Autodesk Inventor part; units mm, degrees
(part 7 of 16)
  spline S39 degree 3 poles (-0.3054, 38.2473) (-0.3514, 38.3741) (-0.3956, 38.5015) (-0.4377, 38.6297) (-0.4605, 38.6989) (-0.4826, 38.7684) (-0.5042, 38.838) (-0.5246, 38.904) (-0.5444, 38.9701) (-0.5636, 39.0364) (-0.5817, 39.099) (-0.5993, 39.1617) (-0.6163, 39.2246) (-0.6323, 39.2837) (-0.6478, 39.3429) (-0.6627, 39.4023) (-0.6767, 39.458) (-0.6902, 39.5137) (-0.7032, 39.5696) (-0.7154, 39.6217) (-0.727, 39.6739) (-0.7382, 39.7262) (-0.7486, 39.7747) (-0.7586, 39.8232) (-0.7681, 39.8719) (-0.7769, 39.9168) (-0.7853, 39.9617) (-0.7932, 40.0067) (-0.8005, 40.0479) (-0.8075, 40.0891) (-0.814, 40.1304) (-0.82, 40.1679) (-0.8256, 40.2054) (-0.8309, 40.243) (-0.8357, 40.2767) (-0.8402, 40.3104) (-0.8443, 40.3442) (-0.8497, 40.3889) (-0.8545, 40.4336) (-0.859, 40.4784) (-0.86, 40.4884) (-0.8609, 40.4984) (-0.862, 40.5084) (-0.8631, 40.5182) (-0.8642, 40.528) (-0.8655, 40.5378) (-0.8667, 40.5473) (-0.868, 40.5568) (-0.8694, 40.5664) (-0.8707, 40.5757) (-0.8722, 40.585) (-0.8737, 40.5944) (-0.8752, 40.6035) (-0.8768, 40.6126) (-0.8785, 40.6217) (-0.8801, 40.6307) (-0.8819, 40.6397) (-0.8837, 40.6486) (-0.8856, 40.6574) (-0.8875, 40.6662) (-0.8895, 40.675) (-0.8915, 40.6837) (-0.8937, 40.6923) (-0.8959, 40.701) (-0.8981, 40.7096) (-0.9005, 40.7181) (-0.9029, 40.7267) (-0.9054, 40.7352) (-0.908, 40.7437) (-0.9107, 40.7522) (-0.9135, 40.7608) (-0.9164, 40.7693) (-0.9194, 40.7777) (-0.9225, 40.7864) (-0.9257, 40.7949) (-0.9292, 40.8034) (-0.9327, 40.8121) (-0.9363, 40.8208) (-0.9402, 40.8294) (-0.9442, 40.8383) (-0.9484, 40.8472) (-0.9529, 40.8559) (-0.9576, 40.8651) (-0.9625, 40.8742) (-0.9676, 40.8832) (-0.9731, 40.8928) (-0.9789, 40.9022) (-0.985, 40.9115) (-0.9917, 40.9215) (-0.9986, 40.9313) (-1.006, 40.9409) (-1.014, 40.9514) (-1.0225, 40.9616) (-1.0314, 40.9715) (-1.0413, 40.9825) (-1.0518, 40.993) (-1.0627, 41.003) (-1.075, 41.0142) (-1.0879, 41.0248) (-1.1014, 41.0346) (-1.1165, 41.0456) (-1.1324, 41.0557) (-1.1488, 41.0646) (-1.1671, 41.0746) (-1.186, 41.0832) (-1.2056, 41.0905) (-1.2267, 41.0983) (-1.2485, 41.1045) (-1.2707, 41.1087) (-1.2918, 41.1127) (-1.3133, 41.1148) (-1.3348, 41.1166) (-1.4411, 41.1253) (-1.5477, 41.1251) (-1.654, 41.13) (-1.7604, 41.135) (-1.8665, 41.1451) (-1.9731, 41.1463) (-1.9947, 41.1465) (-2.0162, 41.1464) (-2.0377, 41.1444) (-2.0601, 41.1423) (-2.0824, 41.1381) (-2.1042, 41.1323) (-2.1243, 41.1269) (-2.144, 41.1201) (-2.1631, 41.1118) (-2.1803, 41.1044) (-2.197, 41.0959) (-2.2131, 41.0863) (-2.2274, 41.0778) (-2.2413, 41.0685) (-2.2546, 41.0585) (-2.2664, 41.0495) (-2.2778, 41.04) (-2.2887, 41.03) (-2.2985, 41.021) (-2.3078, 41.0116) (-2.3169, 41.0019) (-2.325, 40.993) (-2.3329, 40.9839) (-2.3404, 40.9745) (-2.3473, 40.9659) (-2.354, 40.957) (-2.3604, 40.948) (-2.3663, 40.9396) (-2.3721, 40.9309) (-2.3776, 40.9222) (-2.3828, 40.9139) (-2.3878, 40.9055) (-2.3927, 40.897) (-2.3973, 40.8888) (-2.4018, 40.8805) (-2.4061, 40.8721) (-2.4103, 40.864) (-2.4143, 40.8558) (-2.4182, 40.8475) (-2.422, 40.8393) (-2.4256, 40.8311) (-2.4292, 40.8229) (-2.4327, 40.8147) (-2.4361, 40.8064) (-2.4393, 40.7982) (-2.4426, 40.7899) (-2.4457, 40.7816) (-2.4487, 40.7732) (-2.4517, 40.7648) (-2.4547, 40.7564) (-2.4575, 40.7479) (-2.4603, 40.7394) (-2.463, 40.7308) (-2.4657, 40.7222) (-2.4684, 40.7135) (-2.4709, 40.7047) (-2.4734, 40.6959) (-2.476, 40.687) (-2.4784, 40.6781) (-2.4807, 40.6691) (-2.4831, 40.66) (-2.4854, 40.6508) (-2.4876, 40.6417) (-2.4899, 40.6323) (-2.4921, 40.6229) (-2.4942, 40.6135) (-2.4963, 40.6039) (-2.4984, 40.5943) (-2.5003, 40.5847) (-2.5023, 40.5748) (-2.5042, 40.5649) (-2.5062, 40.555) (-2.5147, 40.5109) (-2.5237, 40.4668) (-2.5332, 40.4228) (-2.5405, 40.3895) (-2.5481, 40.3563) (-2.5559, 40.3232) (-2.5647, 40.2863) (-2.5738, 40.2495) (-2.5832, 40.2127) (-2.5935, 40.1722) (-2.6043, 40.1318) (-2.6154, 40.0915) (-2.6275, 40.0474) (-2.64, 40.0034) (-2.6529, 39.9596) (-2.6669, 39.912) (-2.6814, 39.8646) (-2.6962, 39.8173) (-2.7122, 39.7662) (-2.7287, 39.7154) (-2.7456, 39.6646) (-2.7637, 39.6102) (-2.7823, 39.5559) (-2.8014, 39.5018) (-2.8218, 39.4441) (-2.8428, 39.3865) (-2.8642, 39.3291) (-2.887, 39.2681) (-2.9103, 39.2073) (-2.9342, 39.1467) (-2.9594, 39.0825) (-2.9853, 39.0185) (-3.0117, 38.9547) (-3.0396, 38.8873) (-3.0681, 38.8202) (-3.0972, 38.7534) (-3.1511, 38.6297) (-3.2069, 38.5069) (-3.2645, 38.385) knots 0 0 0 0 0.057795 0.057795 0.057795 0.089038 0.089038 0.089038 0.118617 0.118617 0.118617 0.14653 0.14653 0.14653 0.172778 0.172778 0.172778 0.19736 0.19736 0.19736 0.220277 0.220277 0.220277 0.241529 0.241529 0.241529 0.261115 0.261115 0.261115 0.279036 0.279036 0.279036 0.295292 0.295292 0.295292 0.309882 0.309882 0.309882 0.329164 0.329164 0.329164 0.333477 0.333477 0.333477 0.337694 0.337694 0.337694 0.34182 0.34182 0.34182 0.345864 0.345864 0.345864 0.349834 0.349834 0.349834 0.353742 0.353742 0.353742 0.3576 0.3576 0.3576 0.361424 0.361424 0.361424 0.365232 0.365232 0.365232 0.369048 0.369048 0.369048 0.372899 0.372899 0.372899 0.376819 0.376819 0.376819 0.380853 0.380853 0.380853 0.385052 0.385052 0.385052 0.389482 0.389482 0.389482 0.394225 0.394225 0.394225 0.399381 0.399381 0.399381 0.405067 0.405067 0.405067 0.411413 0.411413 0.411413 0.418548 0.418548 0.418548 0.426565 0.426565 0.426565 0.435472 0.435472 0.435472 0.445133 0.445133 0.445133 0.45436 0.45436 0.45436 0.5 0.5 0.5 0.54564 0.54564 0.54564 0.554867 0.554867 0.554867 0.564528 0.564528 0.564528 0.573435 0.573435 0.573435 0.581452 0.581452 0.581452 0.588587 0.588587 0.588587 0.594933 0.594933 0.594933 0.600619 0.600619 0.600619 0.605775 0.605775 0.605775 0.610518 0.610518 0.610518 0.614948 0.614948 0.614948 0.619147 0.619147 0.619147 0.623181 0.623181 0.623181 0.627101 0.627101 0.627101 0.630952 0.630952 0.630952 0.634768 0.634768 0.634768 0.638576 0.638576 0.638576 0.6424 0.6424 0.6424 0.646258 0.646258 0.646258 0.650166 0.650166 0.650166 0.654136 0.654136 0.654136 0.65818 0.65818 0.65818 0.662306 0.662306 0.662306 0.666523 0.666523 0.666523 0.670836 0.670836 0.670836 0.690118 0.690118 0.690118 0.704708 0.704708 0.704708 0.720964 0.720964 0.720964 0.738885 0.738885 0.738885 0.758471 0.758471 0.758471 0.779723 0.779723 0.779723 0.80264 0.80264 0.80264 0.827222 0.827222 0.827222 0.85347 0.85347 0.85347 0.881383 0.881383 0.881383 0.910962 0.910962 0.910962 0.942205 0.942205 0.942205 1 1 1 1
  arc A241 (-0.3054, 38.2473) -> (0.8544, 38.2541) centre (0.0435, 77.6158) ccw
  spline S40 degree 3 poles (3.8116, 38.4265) (3.7526, 38.5478) (3.6954, 38.6699) (3.6401, 38.7929) (3.6102, 38.8594) (3.5809, 38.9262) (3.5522, 38.9932) (3.525, 39.0567) (3.4984, 39.1204) (3.4724, 39.1843) (3.4478, 39.2446) (3.4238, 39.3051) (3.4003, 39.3659) (3.3782, 39.423) (3.3566, 39.4803) (3.3355, 39.5379) (3.3158, 39.5917) (3.2965, 39.6458) (3.2778, 39.7) (3.2603, 39.7505) (3.2432, 39.8012) (3.2266, 39.852) (3.2112, 39.8992) (3.1962, 39.9464) (3.1816, 39.9938) (3.1682, 40.0375) (3.1552, 40.0813) (3.1426, 40.1253) (3.131, 40.1655) (3.1198, 40.2057) (3.1089, 40.2461) (3.0991, 40.2828) (3.0896, 40.3195) (3.0804, 40.3563) (3.0721, 40.3893) (3.0642, 40.4224) (3.0565, 40.4556) (3.0465, 40.4995) (3.037, 40.5434) (3.0279, 40.5875) (3.0259, 40.5974) (3.0238, 40.6072) (3.0217, 40.6171) (3.0196, 40.6267) (3.0175, 40.6363) (3.0152, 40.6459) (3.013, 40.6552) (3.0107, 40.6646) (3.0084, 40.6739) (3.006, 40.6831) (3.0036, 40.6922) (3.0011, 40.7013) (2.9987, 40.7102) (2.9961, 40.7191) (2.9935, 40.728) (2.9909, 40.7368) (2.9882, 40.7455) (2.9855, 40.7542) (2.9827, 40.7627) (2.9799, 40.7713) (2.9769, 40.7798) (2.974, 40.7882) (2.971, 40.7966) (2.9679, 40.805) (2.9648, 40.8133) (2.9615, 40.8216) (2.9582, 40.8298) (2.9549, 40.8381) (2.9514, 40.8463) (2.9478, 40.8544) (2.9442, 40.8626) (2.9404, 40.8708) (2.9365, 40.8789) (2.9325, 40.8871) (2.9284, 40.8953) (2.9241, 40.9034) (2.9197, 40.9117) (2.9152, 40.92) (2.9104, 40.9281) (2.9055, 40.9366) (2.9004, 40.9449) (2.895, 40.9531) (2.8894, 40.9618) (2.8836, 40.9704) (2.8775, 40.9787) (2.871, 40.9877) (2.8643, 40.9965) (2.8572, 41.005) (2.8496, 41.0143) (2.8416, 41.0234) (2.8334, 41.0321) (2.8242, 41.0417) (2.8147, 41.051) (2.8049, 41.0599) (2.7938, 41.0698) (2.7823, 41.0791) (2.7704, 41.0879) (2.757, 41.0978) (2.7431, 41.107) (2.7286, 41.1153) (2.7124, 41.1247) (2.6956, 41.133) (2.6784, 41.1402) (2.6592, 41.1482) (2.6394, 41.1548) (2.6192, 41.16) (2.5973, 41.1656) (2.575, 41.1695) (2.5525, 41.1713) (2.5311, 41.1731) (2.5095, 41.1729) (2.488, 41.1725) (2.3814, 41.1701) (2.2754, 41.1587) (2.1691, 41.1525) (2.0628, 41.1463) (1.9562, 41.1453) (1.85, 41.1353) (1.8286, 41.1333) (1.8071, 41.1309) (1.786, 41.1266) (1.7639, 41.1222) (1.7422, 41.1157) (1.7211, 41.1076) (1.7017, 41.1002) (1.6828, 41.0913) (1.6647, 41.0811) (1.6483, 41.072) (1.6326, 41.0617) (1.6176, 41.0506) (1.6043, 41.0406) (1.5915, 41.0299) (1.5793, 41.0185) (1.5685, 41.0084) (1.5582, 40.9977) (1.5484, 40.9866) (1.5396, 40.9767) (1.5312, 40.9664) (1.5233, 40.9557) (1.5161, 40.9461) (1.5092, 40.9362) (1.5027, 40.9261) (1.4967, 40.9167) (1.491, 40.9072) (1.4856, 40.8976) (1.4806, 40.8886) (1.4758, 40.8794) (1.4712, 40.8701) (1.4669, 40.8613) (1.4627, 40.8525) (1.4588, 40.8435) (1.4551, 40.8348) (1.4515, 40.8261) (1.4481, 40.8174) (1.4448, 40.8088) (1.4416, 40.8002) (1.4386, 40.7916) (1.4357, 40.7831) (1.4329, 40.7745) (1.4303, 40.766) (1.4276, 40.7575) (1.4252, 40.7489) (1.4228, 40.7403) (1.4204, 40.7318) (1.4182, 40.7232) (1.416, 40.7145) (1.4139, 40.7059) (1.4119, 40.6972) (1.41, 40.6885) (1.408, 40.6797) (1.4062, 40.6708) (1.4045, 40.662) (1.4027, 40.6531) (1.4011, 40.6441) (1.3995, 40.6351) (1.398, 40.626) (1.3965, 40.6168) (1.3951, 40.6077) (1.3937, 40.5983) (1.3923, 40.589) (1.3911, 40.5796) (1.3898, 40.5701) (1.3886, 40.5605) (1.3875, 40.551) (1.3864, 40.5412) (1.3854, 40.5314) (1.3844, 40.5216) (1.3834, 40.5116) (1.3826, 40.5016) (1.3817, 40.4915) (1.3778, 40.4467) (1.3735, 40.4019) (1.3686, 40.3572) (1.3649, 40.3234) (1.3608, 40.2896) (1.3564, 40.2558) (1.3516, 40.2182) (1.3464, 40.1806) (1.3409, 40.1431) (1.3348, 40.1017) (1.3284, 40.0604) (1.3215, 40.0191) (1.3141, 39.974) (1.3062, 39.929) (1.298, 39.884) (1.289, 39.8353) (1.2796, 39.7866) (1.2698, 39.7379) (1.2593, 39.6855) (1.2482, 39.6332) (1.2367, 39.581) (1.2243, 39.525) (1.2115, 39.4691) (1.1981, 39.4133) (1.1839, 39.3537) (1.1691, 39.2943) (1.1538, 39.2349) (1.1375, 39.1719) (1.1207, 39.109) (1.1033, 39.0462) (1.0848, 38.9797) (1.0658, 38.9133) (1.0462, 38.8471) (1.0255, 38.7772) (1.0041, 38.7075) (0.9822, 38.638) (0.9416, 38.5094) (0.8989, 38.3814) (0.8544, 38.2541) knots 0 0 0 0 0.057795 0.057795 0.057795 0.089038 0.089038 0.089038 0.118617 0.118617 0.118617 0.14653 0.14653 0.14653 0.172778 0.172778 0.172778 0.19736 0.19736 0.19736 0.220277 0.220277 0.220277 0.241529 0.241529 0.241529 0.261115 0.261115 0.261115 0.279036 0.279036 0.279036 0.295292 0.295292 0.295292 0.309882 0.309882 0.309882 0.329164 0.329164 0.329164 0.333477 0.333477 0.333477 0.337694 0.337694 0.337694 0.34182 0.34182 0.34182 0.345864 0.345864 0.345864 0.349834 0.349834 0.349834 0.353742 0.353742 0.353742 0.3576 0.3576 0.3576 0.361424 0.361424 0.361424 0.365232 0.365232 0.365232 0.369048 0.369048 0.369048 0.372899 0.372899 0.372899 0.376819 0.376819 0.376819 0.380853 0.380853 0.380853 0.385052 0.385052 0.385052 0.389482 0.389482 0.389482 0.394225 0.394225 0.394225 0.399381 0.399381 0.399381 0.405067 0.405067 0.405067 0.411413 0.411413 0.411413 0.418548 0.418548 0.418548 0.426565 0.426565 0.426565 0.435472 0.435472 0.435472 0.445133 0.445133 0.445133 0.45436 0.45436 0.45436 0.5 0.5 0.5 0.54564 0.54564 0.54564 0.554867 0.554867 0.554867 0.564528 0.564528 0.564528 0.573435 0.573435 0.573435 0.581452 0.581452 0.581452 0.588587 0.588587 0.588587 0.594933 0.594933 0.594933 0.600619 0.600619 0.600619 0.605775 0.605775 0.605775 0.610518 0.610518 0.610518 0.614948 0.614948 0.614948 0.619147 0.619147 0.619147 0.623181 0.623181 0.623181 0.627101 0.627101 0.627101 0.630952 0.630952 0.630952 0.634768 0.634768 0.634768 0.638576 0.638576 0.638576 0.6424 0.6424 0.6424 0.646258 0.646258 0.646258 0.650166 0.650166 0.650166 0.654136 0.654136 0.654136 0.65818 0.65818 0.65818 0.662306 0.662306 0.662306 0.666523 0.666523 0.666523 0.670836 0.670836 0.670836 0.690118 0.690118 0.690118 0.704708 0.704708 0.704708 0.720964 0.720964 0.720964 0.738885 0.738885 0.738885 0.758471 0.758471 0.758471 0.779723 0.779723 0.779723 0.80264 0.80264 0.80264 0.827222 0.827222 0.827222 0.85347 0.85347 0.85347 0.881383 0.881383 0.881383 0.910962 0.910962 0.910962 0.942205 0.942205 0.942205 1 1 1 1
  arc A242 (3.8116, 38.4265) -> (4.9644, 38.5545) centre (0.0435, 77.6158) ccw
  spline S41 degree 3 poles (7.8874, 39.0351) (7.816, 39.1495) (7.7463, 39.265) (7.6785, 39.3816) (7.6418, 39.4446) (7.6057, 39.5079) (7.5701, 39.5716) (7.5365, 39.6318) (7.5034, 39.6924) (7.4708, 39.7532) (7.4401, 39.8107) (7.4098, 39.8684) (7.3801, 39.9263) (7.3522, 39.9808) (7.3247, 40.0356) (7.2977, 40.0906) (7.2725, 40.1421) (7.2477, 40.1938) (7.2233, 40.2457) (7.2006, 40.2942) (7.1784, 40.3428) (7.1565, 40.3916) (7.1363, 40.4369) (7.1164, 40.4823) (7.097, 40.528) (7.0791, 40.57) (7.0616, 40.6122) (7.0444, 40.6546) (7.0287, 40.6933) (7.0133, 40.7322) (6.9983, 40.7713) (6.9847, 40.8067) (6.9714, 40.8422) (6.9584, 40.8778) (6.9468, 40.9098) (6.9354, 40.9419) (6.9243, 40.9741) (6.9097, 41.0167) (6.8957, 41.0594) (6.8821, 41.1023) (6.879, 41.1119) (6.876, 41.1215) (6.8728, 41.1311) (6.8698, 41.1404) (6.8666, 41.1497) (6.8633, 41.159) (6.8602, 41.1681) (6.8569, 41.1772) (6.8536, 41.1862) (6.8503, 41.1951) (6.847, 41.2039) (6.8435, 41.2127) (6.8402, 41.2213) (6.8367, 41.2299) (6.8332, 41.2385) (6.8297, 41.2469) (6.8261, 41.2553) (6.8224, 41.2636) (6.8188, 41.2719) (6.8151, 41.2801) (6.8113, 41.2882) (6.8075, 41.2963) (6.8036, 41.3043) (6.7996, 41.3123) (6.7957, 41.3203) (6.7916, 41.3282) (6.7874, 41.336) (6.7832, 41.3439) (6.7789, 41.3517) (6.7745, 41.3594) (6.77, 41.3672) (6.7654, 41.3749) (6.7607, 41.3825) (6.7559, 41.3903) (6.7509, 41.398) (6.7458, 41.4056) (6.7406, 41.4134) (6.7352, 41.4211) (6.7296, 41.4287) (6.7238, 41.4366) (6.7179, 41.4444) (6.7117, 41.452) (6.7052, 41.4601) (6.6985, 41.468) (6.6916, 41.4757) (6.6842, 41.4839) (6.6766, 41.4919) (6.6687, 41.4997) (6.6601, 41.5081) (6.6513, 41.5163) (6.6421, 41.5241) (6.632, 41.5328) (6.6216, 41.541) (6.6109, 41.5488) (6.5989, 41.5575) (6.5865, 41.5656) (6.5737, 41.5731) (6.5593, 41.5815) (6.5445, 41.5892) (6.5293, 41.596) (6.5122, 41.6036) (6.4946, 41.6101) (6.4767, 41.6155) (6.4567, 41.6214) (6.4364, 41.6259) (6.4158, 41.6289) (6.3934, 41.6322) (6.3708, 41.6337) (6.3483, 41.6332) (6.3268, 41.6327) (6.3053, 41.6304) (6.2839, 41.6276) (6.1782, 41.6141) (6.0739, 41.5917) (5.9689, 41.5744) (5.8638, 41.5571) (5.7579, 41.545) (5.6534, 41.524) (5.6323, 41.5197) (5.6112, 41.5151) (5.5906, 41.5087) (5.5691, 41.5019) (5.5482, 41.4932) (5.5281, 41.483) (5.5095, 41.4735) (5.4917, 41.4628) (5.4747, 41.4507) (5.4594, 41.4399) (5.4448, 41.4281) (5.4311, 41.4154) (5.4188, 41.4041) (5.4072, 41.3921) (5.3963, 41.3795) (5.3866, 41.3683) (5.3775, 41.3567) (5.3689, 41.3446) (5.3612, 41.3338) (5.354, 41.3226) (5.3472, 41.3112) (5.341, 41.3009) (5.3352, 41.2903) (5.3298, 41.2796) (5.3249, 41.2697) (5.3202, 41.2597) (5.3158, 41.2495) (5.3117, 41.24) (5.3079, 41.2304) (5.3043, 41.2207) (5.3009, 41.2115) (5.2978, 41.2022) (5.2948, 41.1929) (5.292, 41.1839) (5.2893, 41.1748) (5.2869, 41.1658) (5.2845, 41.1569) (5.2823, 41.1481) (5.2802, 41.1391) (5.2782, 41.1304) (5.2763, 41.1216) (5.2745, 41.1128) (5.2728, 41.104) (5.2712, 41.0953) (5.2698, 41.0865) (5.2683, 41.0777) (5.267, 41.0689) (5.2658, 41.0601) (5.2645, 41.0513) (5.2634, 41.0424) (5.2624, 41.0336) (5.2614, 41.0246) (5.2605, 41.0157) (5.2598, 41.0067) (5.2589, 40.9976) (5.2582, 40.9885) (5.2576, 40.9794) (5.257, 40.9702) (5.2565, 40.9609) (5.2561, 40.9517) (5.2556, 40.9423) (5.2553, 40.9328) (5.255, 40.9234) (5.2548, 40.9138) (5.2546, 40.9041) (5.2545, 40.8945) (5.2544, 40.8847) (5.2544, 40.8748) (5.2545, 40.865) (5.2545, 40.8549) (5.2547, 40.8449) (5.2549, 40.8348) (5.2557, 40.7898) (5.2561, 40.7448) (5.2559, 40.6998) (5.2558, 40.6658) (5.2552, 40.6317) (5.2544, 40.5977) (5.2535, 40.5598) (5.2523, 40.5219) (5.2507, 40.484) (5.249, 40.4422) (5.2469, 40.4004) (5.2445, 40.3587) (5.2418, 40.313) (5.2387, 40.2674) (5.2352, 40.2219) (5.2314, 40.1724) (5.2271, 40.123) (5.2224, 40.0736) (5.2174, 40.0204) (5.2118, 39.9672) (5.2059, 39.9141) (5.1994, 39.8571) (5.1925, 39.8001) (5.1851, 39.7432) (5.1771, 39.6825) (5.1686, 39.6218) (5.1596, 39.5613) (5.15, 39.4968) (5.1398, 39.4325) (5.1291, 39.3682) (5.1177, 39.3002) (5.1057, 39.2322) (5.0931, 39.1643) (5.0798, 39.0926) (5.0659, 39.0211) (5.0513, 38.9496) (5.0244, 38.8175) (4.9953, 38.6858) (4.9644, 38.5545) knots 0 0 0 0 0.057795 0.057795 0.057795 0.089038 0.089038 0.089038 0.118617 0.118617 0.118617 0.14653 0.14653 0.14653 0.172778 0.172778 0.172778 0.19736 0.19736 0.19736 0.220277 0.220277 0.220277 0.241529 0.241529 0.241529 0.261115 0.261115 0.261115 0.279036 0.279036 0.279036 0.295292 0.295292 0.295292 0.309882 0.309882 0.309882 0.329164 0.329164 0.329164 0.333477 0.333477 0.333477 0.337694 0.337694 0.337694 0.34182 0.34182 0.34182 0.345864 0.345864 0.345864 0.349834 0.349834 0.349834 0.353742 0.353742 0.353742 0.3576 0.3576 0.3576 0.361424 0.361424 0.361424 0.365232 0.365232 0.365232 0.369048 0.369048 0.369048 0.372899 0.372899 0.372899 0.376819 0.376819 0.376819 0.380853 0.380853 0.380853 0.385052 0.385052 0.385052 0.389482 0.389482 0.389482 0.394225 0.394225 0.394225 0.399381 0.399381 0.399381 0.405067 0.405067 0.405067 0.411413 0.411413 0.411413 0.418548 0.418548 0.418548 0.426565 0.426565 0.426565 0.435472 0.435472 0.435472 0.445133 0.445133 0.445133 0.45436 0.45436 0.45436 0.5 0.5 0.5 0.54564 0.54564 0.54564 0.554867 0.554867 0.554867 0.564528 0.564528 0.564528 0.573435 0.573435 0.573435 0.581452 0.581452 0.581452 0.588587 0.588587 0.588587 0.594933 0.594933 0.594933 0.600619 0.600619 0.600619 0.605775 0.605775 0.605775 0.610518 0.610518 0.610518 0.614948 0.614948 0.614948 0.619147 0.619147 0.619147 0.623181 0.623181 0.623181 0.627101 0.627101 0.627101 0.630952 0.630952 0.630952 0.634768 0.634768 0.634768 0.638576 0.638576 0.638576 0.6424 0.6424 0.6424 0.646258 0.646258 0.646258 0.650166 0.650166 0.650166 0.654136 0.654136 0.654136 0.65818 0.65818 0.65818 0.662306 0.662306 0.662306 0.666523 0.666523 0.666523 0.670836 0.670836 0.670836 0.690118 0.690118 0.690118 0.704708 0.704708 0.704708 0.720964 0.720964 0.720964 0.738885 0.738885 0.738885 0.758471 0.758471 0.758471 0.779723 0.779723 0.779723 0.80264 0.80264 0.80264 0.827222 0.827222 0.827222 0.85347 0.85347 0.85347 0.881383 0.881383 0.881383 0.910962 0.910962 0.910962 0.942205 0.942205 0.942205 1 1 1 1
  arc A243 (7.8874, 39.0351) -> (9.0204, 39.2829) centre (0.0435, 77.6158) ccw
  spline S42 degree 3 poles (11.8772, 40.0663) (11.7942, 40.1727) (11.7129, 40.2802) (11.6332, 40.3891) (11.5902, 40.4479) (11.5476, 40.5071) (11.5056, 40.5667) (11.4658, 40.6231) (11.4266, 40.6799) (11.3878, 40.737) (11.3512, 40.7909) (11.3151, 40.8451) (11.2795, 40.8997) (11.246, 40.951) (11.213, 41.0025) (11.1804, 41.0544) (11.1499, 41.103) (11.1198, 41.1518) (11.0902, 41.201) (11.0626, 41.2467) (11.0354, 41.2928) (11.0086, 41.339) (10.9837, 41.382) (10.9592, 41.4251) (10.9351, 41.4684) (10.9129, 41.5084) (10.891, 41.5485) (10.8696, 41.5889) (10.8499, 41.6258) (10.8305, 41.6628) (10.8115, 41.7001) (10.7943, 41.7339) (10.7774, 41.7678) (10.7607, 41.8019) (10.7458, 41.8325) (10.7311, 41.8632) (10.7167, 41.8941) (10.6977, 41.9349) (10.6794, 41.976) (10.6613, 42.0172) (10.6573, 42.0264) (10.6532, 42.0356) (10.6491, 42.0448) (10.6451, 42.0538) (10.6409, 42.0627) (10.6367, 42.0716) (10.6326, 42.0803) (10.6285, 42.089) (10.6242, 42.0976) (10.62, 42.1061) (10.6158, 42.1145) (10.6115, 42.1229) (10.6072, 42.1311) (10.6029, 42.1393) (10.5984, 42.1475) (10.5941, 42.1555) (10.5897, 42.1634) (10.5851, 42.1714) (10.5807, 42.1792) (10.5761, 42.1869) (10.5715, 42.1947) (10.5669, 42.2023) (10.5622, 42.2099) (10.5574, 42.2174) (10.5526, 42.2249) (10.5477, 42.2323) (10.5427, 42.2397) (10.5377, 42.2471) (10.5326, 42.2544) (10.5274, 42.2616) (10.5222, 42.2689) (10.5168, 42.2761) (10.5113, 42.2832) (10.5057, 42.2904) (10.5, 42.2975) (10.4941, 42.3046) (10.4881, 42.3118) (10.4819, 42.3189) (10.4756, 42.3259) (10.469, 42.3331) (10.4622, 42.3402) (10.4553, 42.3472) (10.448, 42.3545) (10.4405, 42.3616) (10.4329, 42.3686) (10.4246, 42.376) (10.4162, 42.3832) (10.4076, 42.3901) (10.3981, 42.3976) (10.3885, 42.4048) (10.3786, 42.4116) (10.3676, 42.4191) (10.3564, 42.4262) (10.3449, 42.4328) (10.3321, 42.4402) (10.3189, 42.447) (10.3054, 42.4531) (10.2902, 42.46) (10.2747, 42.4661) (10.2588, 42.4712) (10.241, 42.477) (10.2229, 42.4817) (10.2045, 42.4851) (10.184, 42.489) (10.1633, 42.4913) (10.1425, 42.4921) (10.1199, 42.4931) (10.0973, 42.4922) (10.0749, 42.4894) (10.0536, 42.4866) (10.0325, 42.482) (10.0115, 42.4771) (9.9078, 42.4526) (9.8065, 42.4194) (9.7038, 42.3912) (9.6011, 42.3631) (9.497, 42.3399) (9.3953, 42.3081) (9.3747, 42.3016) (9.3542, 42.2948) (9.3345, 42.2863) (9.3138, 42.2774) (9.2939, 42.2665) (9.2749, 42.2542) (9.2575, 42.2429) (9.2408, 42.2303) (9.2252, 42.2166) (9.2111, 42.2042) (9.1979, 42.1909) (9.1855, 42.1769) (9.1746, 42.1644) (9.1643, 42.1512) (9.1547, 42.1376) (9.1463, 42.1254) (9.1384, 42.1128) (9.1311, 42.0999) (9.1246, 42.0884) (9.1185, 42.0766) (9.113, 42.0645) (9.1079, 42.0536) (9.1033, 42.0425) (9.099, 42.0312) (9.0951, 42.0209) (9.0915, 42.0104) (9.0882, 41.9998) (9.0852, 41.9899) (9.0824, 41.98) (9.0798, 41.97) (9.0774, 41.9605) (9.0753, 41.9509) (9.0733, 41.9413) (9.0714, 41.9321) (9.0697, 41.9228) (9.0682, 41.9135) (9.0668, 41.9045) (9.0655, 41.8954) (9.0643, 41.8863) (9.0632, 41.8774) (9.0623, 41.8685) (9.0615, 41.8595) (9.0607, 41.8507) (9.06, 41.8418) (9.0595, 41.8329) (9.0589, 41.824) (9.0585, 41.8152) (9.0583, 41.8063) (9.058, 41.7974) (9.0578, 41.7884) (9.0577, 41.7795) (9.0577, 41.7705) (9.0577, 41.7615) (9.0579, 41.7525) (9.058, 41.7434) (9.0583, 41.7343) (9.0586, 41.7252) (9.059, 41.7159) (9.0594, 41.7066) (9.06, 41.6974) (9.0605, 41.688) (9.0612, 41.6786) (9.0619, 41.6692) (9.0626, 41.6596) (9.0635, 41.65) (9.0644, 41.6404) (9.0653, 41.6306) (9.0663, 41.6208) (9.0674, 41.611) (9.0686, 41.601) (9.0698, 41.591) (9.071, 41.581) (9.0765, 41.5364) (9.0816, 41.4917) (9.0861, 41.4469) (9.0895, 41.413) (9.0926, 41.3791) (9.0953, 41.3452) (9.0984, 41.3074) (9.1011, 41.2695) (9.1036, 41.2317) (9.1062, 41.1899) (9.1085, 41.1482) (9.1104, 41.1064) (9.1125, 41.0607) (9.1142, 41.0151) (9.1154, 40.9694) (9.1168, 40.9198) (9.1178, 40.8702) (9.1183, 40.8206) (9.1188, 40.7672) (9.1189, 40.7137) (9.1185, 40.6602) (9.1181, 40.6028) (9.1171, 40.5455) (9.1156, 40.4881) (9.1141, 40.4269) (9.112, 40.3657) (9.1093, 40.3045) (9.1065, 40.2394) (9.1031, 40.1744) (9.0992, 40.1094) (9.095, 40.0405) (9.0902, 39.9716) (9.0847, 39.9028) (9.079, 39.8301) (9.0726, 39.7575) (9.0656, 39.6849) (9.0526, 39.5507) (9.0375, 39.4166) (9.0204, 39.2829) knots 0 0 0 0 0.057795 0.057795 0.057795 0.089038 0.089038 0.089038 0.118617 0.118617 0.118617 0.14653 0.14653 0.14653 0.172778 0.172778 0.172778 0.19736 0.19736 0.19736 0.220277 0.220277 0.220277 0.241529 0.241529 0.241529 0.261115 0.261115 0.261115 0.279036 0.279036 0.279036 0.295292 0.295292 0.295292 0.309882 0.309882 0.309882 0.329164 0.329164 0.329164 0.333477 0.333477 0.333477 0.337694 0.337694 0.337694 0.34182 0.34182 0.34182 0.345864 0.345864 0.345864 0.349834 0.349834 0.349834 0.353742 0.353742 0.353742 0.3576 0.3576 0.3576 0.361424 0.361424 0.361424 0.365232 0.365232 0.365232 0.369048 0.369048 0.369048 0.372899 0.372899 0.372899 0.376819 0.376819 0.376819 0.380853 0.380853 0.380853 0.385052 0.385052 0.385052 0.389482 0.389482 0.389482 0.394225 0.394225 0.394225 0.399381 0.399381 0.399381 0.405067 0.405067 0.405067 0.411413 0.411413 0.411413 0.418548 0.418548 0.418548 0.426565 0.426565 0.426565 0.435472 0.435472 0.435472 0.445133 0.445133 0.445133 0.45436 0.45436 0.45436 0.5 0.5 0.5 0.54564 0.54564 0.54564 0.554867 0.554867 0.554867 0.564528 0.564528 0.564528 0.573435 0.573435 0.573435 0.581452 0.581452 0.581452 0.588587 0.588587 0.588587 0.594933 0.594933 0.594933 0.600619 0.600619 0.600619 0.605775 0.605775 0.605775 0.610518 0.610518 0.610518 0.614948 0.614948 0.614948 0.619147 0.619147 0.619147 0.623181 0.623181 0.623181 0.627101 0.627101 0.627101 0.630952 0.630952 0.630952 0.634768 0.634768 0.634768 0.638576 0.638576 0.638576 0.6424 0.6424 0.6424 0.646258 0.646258 0.646258 0.650166 0.650166 0.650166 0.654136 0.654136 0.654136 0.65818 0.65818 0.65818 0.662306 0.662306 0.662306 0.666523 0.666523 0.666523 0.670836 0.670836 0.670836 0.690118 0.690118 0.690118 0.704708 0.704708 0.704708 0.720964 0.720964 0.720964 0.738885 0.738885 0.738885 0.758471 0.758471 0.758471 0.779723 0.779723 0.779723 0.80264 0.80264 0.80264 0.827222 0.827222 0.827222 0.85347 0.85347 0.85347 0.881383 0.881383 0.881383 0.910962 0.910962 0.910962 0.942205 0.942205 0.942205 1 1 1 1
  arc A244 (11.8772, 40.0663) -> (12.9781, 40.4312) centre (0.0435, 77.6158) ccw
  spline S43 degree 3 poles (15.7373, 41.509) (15.6437, 41.6061) (15.5516, 41.7045) (15.461, 41.8045) (15.412, 41.8585) (15.3635, 41.9129) (15.3155, 41.9678) (15.2701, 42.0197) (15.2251, 42.0721) (15.1806, 42.1248) (15.1385, 42.1746) (15.097, 42.2248) (15.0559, 42.2753) (15.0172, 42.3228) (14.9789, 42.3706) (14.9411, 42.4188) (14.9057, 42.4639) (14.8707, 42.5094) (14.8361, 42.5551) (14.8038, 42.5978) (14.7719, 42.6407) (14.7404, 42.6839) (14.7112, 42.724) (14.6824, 42.7643) (14.6539, 42.8049) (14.6276, 42.8423) (14.6017, 42.88) (14.5761, 42.9178) (14.5527, 42.9525) (14.5295, 42.9873) (14.5068, 43.0224) (14.4861, 43.0542) (14.4657, 43.0862) (14.4456, 43.1184) (14.4275, 43.1472) (14.4097, 43.1762) (14.3922, 43.2054) (14.3691, 43.244) (14.3465, 43.2829) (14.3242, 43.322) (14.3192, 43.3308) (14.3142, 43.3395) (14.3092, 43.3482) (14.3042, 43.3567) (14.2992, 43.3652) (14.2941, 43.3736) (14.2891, 43.3818) (14.284, 43.39) (14.2789, 43.3982) (14.2739, 43.4062) (14.2688, 43.4141) (14.2636, 43.422) (14.2585, 43.4297) (14.2533, 43.4374) (14.2481, 43.445) (14.2429, 43.4526) (14.2377, 43.46) (14.2323, 43.4674) (14.2271, 43.4747) (14.2217, 43.482) (14.2163, 43.4892) (14.2109, 43.4963) (14.2055, 43.5033) (14.1999, 43.5103) (14.1944, 43.5173) (14.1888, 43.5242) (14.183, 43.531) (14.1773, 43.5378) (14.1715, 43.5445) (14.1655, 43.5511) (14.1595, 43.5578) (14.1534, 43.5644) (14.1472, 43.5709) (14.1409, 43.5775) (14.1344, 43.584) (14.1279, 43.5904) (14.1211, 43.5969) (14.1142, 43.6034) (14.1072, 43.6096) (14.0999, 43.6162) (14.0925, 43.6225) (14.0848, 43.6287) (14.0768, 43.6352) (14.0686, 43.6415) (14.0603, 43.6476) (14.0513, 43.6542) (14.0422, 43.6604) (14.0329, 43.6664) (14.0227, 43.6729) (14.0124, 43.679) (14.0018, 43.6848) (13.9901, 43.6911) (13.9782, 43.697) (13.9661, 43.7024) (13.9526, 43.7084) (13.9387, 43.7137) (13.9247, 43.7184) (13.9089, 43.7237) (13.8928, 43.7281) (13.8765, 43.7315) (13.8582, 43.7354) (13.8396, 43.7382) (13.821, 43.7397) (13.8002, 43.7414) (13.7794, 43.7415) (13.7586, 43.7402) (13.7361, 43.7387) (13.7136, 43.7356) (13.6917, 43.7304) (13.6707, 43.7254) (13.6503, 43.7186) (13.6299, 43.7115) (13.5293, 43.6763) (13.432, 43.6327) (13.3328, 43.594) (13.2336, 43.5552) (13.1326, 43.5213) (13.0347, 43.479) (13.0149, 43.4705) (12.9953, 43.4616) (12.9765, 43.451) (12.9569, 43.44) (12.9382, 43.4271) (12.9206, 43.4129) (12.9045, 43.3998) (12.8892, 43.3855) (12.8751, 43.3702) (12.8624, 43.3565) (12.8507, 43.3419) (12.8398, 43.3266) (12.8302, 43.313) (12.8214, 43.2989) (12.8133, 43.2843) (12.8061, 43.2713) (12.7996, 43.258) (12.7937, 43.2444) (12.7885, 43.2322) (12.7837, 43.2198) (12.7794, 43.2073) (12.7755, 43.1959) (12.7721, 43.1843) (12.769, 43.1727) (12.7662, 43.162) (12.7637, 43.1512) (12.7616, 43.1403) (12.7596, 43.1302) (12.7578, 43.12) (12.7563, 43.1098) (12.7549, 43.1001) (12.7538, 43.0903) (12.7528, 43.0806) (12.7519, 43.0712) (12.7512, 43.0618) (12.7507, 43.0524) (12.7502, 43.0433) (12.7498, 43.0342) (12.7497, 43.025) (12.7495, 43.016) (12.7495, 43.007) (12.7496, 42.9981) (12.7497, 42.9892) (12.75, 42.9803) (12.7504, 42.9714) (12.7508, 42.9625) (12.7513, 42.9536) (12.752, 42.9447) (12.7526, 42.9358) (12.7534, 42.927) (12.7543, 42.9181) (12.7551, 42.9091) (12.7561, 42.9002) (12.7572, 42.8912) (12.7583, 42.8822) (12.7595, 42.8731) (12.7608, 42.8641) (12.7621, 42.8549) (12.7636, 42.8458) (12.7651, 42.8366) (12.7666, 42.8273) (12.7682, 42.818) (12.7699, 42.8087) (12.7717, 42.7993) (12.7735, 42.7898) (12.7754, 42.7804) (12.7774, 42.7707) (12.7794, 42.7611) (12.7815, 42.7515) (12.7837, 42.7417) (12.786, 42.7319) (12.7882, 42.7221) (12.7984, 42.6782) (12.8081, 42.6343) (12.8173, 42.5903) (12.8242, 42.5569) (12.8308, 42.5235) (12.837, 42.49) (12.8441, 42.4528) (12.8507, 42.4154) (12.8571, 42.378) (12.8641, 42.3368) (12.8707, 42.2955) (12.877, 42.2542) (12.8838, 42.209) (12.8903, 42.1637) (12.8963, 42.1184) (12.9029, 42.0693) (12.909, 42.02) (12.9147, 41.9708) (12.9208, 41.9177) (12.9265, 41.8645) (12.9317, 41.8112) (12.9372, 41.7542) (12.9423, 41.697) (12.9468, 41.6398) (12.9517, 41.5788) (12.956, 41.5177) (12.9598, 41.4565) (12.9638, 41.3915) (12.9672, 41.3265) (12.9701, 41.2614) (12.9731, 41.1924) (12.9755, 41.1235) (12.9773, 41.0545) (12.9792, 40.9816) (12.9804, 40.9087) (12.981, 40.8358) (12.9822, 40.7009) (12.9811, 40.566) (12.9781, 40.4312) knots 0 0 0 0 0.057795 0.057795 0.057795 0.089038 0.089038 0.089038 0.118617 0.118617 0.118617 0.14653 0.14653 0.14653 0.172778 0.172778 0.172778 0.19736 0.19736 0.19736 0.220277 0.220277 0.220277 0.241529 0.241529 0.241529 0.261115 0.261115 0.261115 0.279036 0.279036 0.279036 0.295292 0.295292 0.295292 0.309882 0.309882 0.309882 0.329164 0.329164 0.329164 0.333477 0.333477 0.333477 0.337694 0.337694 0.337694 0.34182 0.34182 0.34182 0.345864 0.345864 0.345864 0.349834 0.349834 0.349834 0.353742 0.353742 0.353742 0.3576 0.3576 0.3576 0.361424 0.361424 0.361424 0.365232 0.365232 0.365232 0.369048 0.369048 0.369048 0.372899 0.372899 0.372899 0.376819 0.376819 0.376819 0.380853 0.380853 0.380853 0.385052 0.385052 0.385052 0.389482 0.389482 0.389482 0.394225 0.394225 0.394225 0.399381 0.399381 0.399381 0.405067 0.405067 0.405067 0.411413 0.411413 0.411413 0.418548 0.418548 0.418548 0.426565 0.426565 0.426565 0.435472 0.435472 0.435472 0.445133 0.445133 0.445133 0.45436 0.45436 0.45436 0.5 0.5 0.5 0.54564 0.54564 0.54564 0.554867 0.554867 0.554867 0.564528 0.564528 0.564528 0.573435 0.573435 0.573435 0.581452 0.581452 0.581452 0.588587 0.588587 0.588587 0.594933 0.594933 0.594933 0.600619 0.600619 0.600619 0.605775 0.605775 0.605775 0.610518 0.610518 0.610518 0.614948 0.614948 0.614948 0.619147 0.619147 0.619147 0.623181 0.623181 0.623181 0.627101 0.627101 0.627101 0.630952 0.630952 0.630952 0.634768 0.634768 0.634768 0.638576 0.638576 0.638576 0.6424 0.6424 0.6424 0.646258 0.646258 0.646258 0.650166 0.650166 0.650166 0.654136 0.654136 0.654136 0.65818 0.65818 0.65818 0.662306 0.662306 0.662306 0.666523 0.666523 0.666523 0.670836 0.670836 0.670836 0.690118 0.690118 0.690118 0.704708 0.704708 0.704708 0.720964 0.720964 0.720964 0.738885 0.738885 0.738885 0.758471 0.758471 0.758471 0.779723 0.779723 0.779723 0.80264 0.80264 0.80264 0.827222 0.827222 0.827222 0.85347 0.85347 0.85347 0.881383 0.881383 0.881383 0.910962 0.910962 0.910962 0.942205 0.942205 0.942205 1 1 1 1
  arc A245 (15.7373, 41.509) -> (16.7941, 41.9869) centre (0.0435, 77.6158) ccw
  spline S44 degree 3 poles (19.4256, 43.3472) (19.3223, 43.434) (19.2204, 43.5223) (19.1198, 43.6122) (19.0655, 43.6608) (19.0115, 43.7099) (18.9581, 43.7594) (18.9074, 43.8064) (18.8572, 43.8537) (18.8074, 43.9015) (18.7605, 43.9466) (18.7139, 43.9922) (18.6677, 44.0381) (18.6243, 44.0813) (18.5812, 44.1249) (18.5386, 44.1689) (18.4987, 44.21) (18.4591, 44.2516) (18.4199, 44.2934) (18.3833, 44.3325) (18.3471, 44.3719) (18.3113, 44.4115) (18.2781, 44.4483) (18.2451, 44.4854) (18.2126, 44.5228) (18.1825, 44.5573) (18.1528, 44.592) (18.1234, 44.627) (18.0965, 44.659) (18.0698, 44.6912) (18.0435, 44.7237) (18.0196, 44.7532) (17.996, 44.7829) (17.9726, 44.8128) (17.9517, 44.8396) (17.9309, 44.8666) (17.9104, 44.8938) (17.8834, 44.9297) (17.8569, 44.9661) (17.8306, 45.0026) (17.8248, 45.0108) (17.8189, 45.019) (17.813, 45.0271) (17.8072, 45.0351) (17.8013, 45.043) (17.7953, 45.0508) (17.7895, 45.0584) (17.7836, 45.0661) (17.7776, 45.0736) (17.7718, 45.081) (17.7659, 45.0884) (17.7599, 45.0957) (17.754, 45.1029) (17.7481, 45.11) (17.7421, 45.117) (17.7362, 45.124) (17.7302, 45.1308) (17.7241, 45.1376) (17.7181, 45.1444) (17.712, 45.151) (17.7059, 45.1576) (17.6998, 45.1641) (17.6936, 45.1705) (17.6874, 45.1769) (17.6811, 45.1832) (17.6748, 45.1895) (17.6684, 45.1957) (17.662, 45.2018) (17.6555, 45.2079) (17.6489, 45.2139) (17.6422, 45.2199) (17.6355, 45.2258) (17.6286, 45.2317) (17.6216, 45.2376) (17.6145, 45.2434) (17.6073, 45.249) (17.5999, 45.2548) (17.5924, 45.2605) (17.5848, 45.266) (17.5768, 45.2717) (17.5688, 45.2773) (17.5605, 45.2826) (17.5519, 45.2883) (17.5431, 45.2937) (17.5341, 45.2989) (17.5246, 45.3044) (17.5148, 45.3097) (17.5049, 45.3146) (17.4941, 45.32) (17.4832, 45.325) (17.4721, 45.3297) (17.4598, 45.3348) (17.4474, 45.3394) (17.4347, 45.3434) (17.4207, 45.348) (17.4063, 45.3519) (17.3919, 45.3551) (17.3756, 45.3587) (17.3591, 45.3614) (17.3426, 45.3631) (17.324, 45.3651) (17.3052, 45.3659) (17.2865, 45.3654) (17.2657, 45.3649) (17.245, 45.3629) (17.2244, 45.3594) (17.2022, 45.3556) (17.1802, 45.3501) (17.1589, 45.3426) (17.1386, 45.3355) (17.1189, 45.3266) (17.0994, 45.3174) (17.003, 45.2719) (16.9108, 45.2183) (16.8163, 45.1694) (16.7217, 45.1206) (16.6247, 45.0763) (16.5318, 45.024) (16.513, 45.0134) (16.4944, 45.0025) (16.4768, 44.99) (16.4585, 44.977) (16.4412, 44.9622) (16.4253, 44.9463) (16.4106, 44.9316) (16.3969, 44.9158) (16.3845, 44.8991) (16.3733, 44.8841) (16.3631, 44.8684) (16.3539, 44.852) (16.3458, 44.8375) (16.3385, 44.8225) (16.332, 44.8072) (16.3262, 44.7935) (16.3211, 44.7796) (16.3167, 44.7655) (16.3127, 44.7528) (16.3092, 44.74) (16.3063, 44.727) (16.3037, 44.7153) (16.3014, 44.7035) (16.2996, 44.6916) (16.2979, 44.6806) (16.2966, 44.6696) (16.2956, 44.6586) (16.2946, 44.6483) (16.294, 44.638) (16.2936, 44.6277) (16.2932, 44.6179) (16.293, 44.6081) (16.2931, 44.5983) (16.2932, 44.5889) (16.2935, 44.5794) (16.2939, 44.57) (16.2944, 44.5609) (16.295, 44.5518) (16.2958, 44.5427) (16.2966, 44.5337) (16.2975, 44.5248) (16.2985, 44.5158) (16.2996, 44.507) (16.3008, 44.4982) (16.3021, 44.4894) (16.3035, 44.4806) (16.3049, 44.4718) (16.3065, 44.4631) (16.308, 44.4543) (16.3097, 44.4455) (16.3115, 44.4368) (16.3133, 44.428) (16.3153, 44.4192) (16.3173, 44.4104) (16.3193, 44.4015) (16.3215, 44.3926) (16.3237, 44.3838) (16.326, 44.3748) (16.3283, 44.3659) (16.3308, 44.3569) (16.3333, 44.3478) (16.3359, 44.3387) (16.3385, 44.3297) (16.3413, 44.3205) (16.3441, 44.3113) (16.3469, 44.3021) (16.3499, 44.2927) (16.3529, 44.2833) (16.356, 44.274) (16.3592, 44.2644) (16.3625, 44.2549) (16.3658, 44.2454) (16.3805, 44.2029) (16.3948, 44.1602) (16.4085, 44.1173) (16.4188, 44.0849) (16.4288, 44.0524) (16.4386, 44.0198) (16.4495, 43.9834) (16.46, 43.947) (16.4702, 43.9104) (16.4815, 43.8702) (16.4924, 43.8298) (16.503, 43.7893) (16.5145, 43.7451) (16.5257, 43.7008) (16.5364, 43.6564) (16.5481, 43.6082) (16.5593, 43.5599) (16.5701, 43.5115) (16.5818, 43.4593) (16.5929, 43.407) (16.6037, 43.3546) (16.6152, 43.2984) (16.6262, 43.2421) (16.6367, 43.1857) (16.6479, 43.1255) (16.6585, 43.0651) (16.6687, 43.0047) (16.6795, 42.9405) (16.6897, 42.8762) (16.6993, 42.8117) (16.7095, 42.7435) (16.7191, 42.6751) (16.7281, 42.6067) (16.7376, 42.5344) (16.7465, 42.462) (16.7547, 42.3896) (16.7699, 42.2556) (16.783, 42.1213) (16.7941, 41.9869) knots 0 0 0 0 0.057795 0.057795 0.057795 0.089038 0.089038 0.089038 0.118617 0.118617 0.118617 0.14653 0.14653 0.14653 0.172778 0.172778 0.172778 0.19736 0.19736 0.19736 0.220277 0.220277 0.220277 0.241529 0.241529 0.241529 0.261115 0.261115 0.261115 0.279036 0.279036 0.279036 0.295292 0.295292 0.295292 0.309882 0.309882 0.309882 0.329164 0.329164 0.329164 0.333477 0.333477 0.333477 0.337694 0.337694 0.337694 0.34182 0.34182 0.34182 0.345864 0.345864 0.345864 0.349834 0.349834 0.349834 0.353742 0.353742 0.353742 0.3576 0.3576 0.3576 0.361424 0.361424 0.361424 0.365232 0.365232 0.365232 0.369048 0.369048 0.369048 0.372899 0.372899 0.372899 0.376819 0.376819 0.376819 0.380853 0.380853 0.380853 0.385052 0.385052 0.385052 0.389482 0.389482 0.389482 0.394225 0.394225 0.394225 0.399381 0.399381 0.399381 0.405067 0.405067 0.405067 0.411413 0.411413 0.411413 0.418548 0.418548 0.418548 0.426565 0.426565 0.426565 0.435472 0.435472 0.435472 0.445133 0.445133 0.445133 0.45436 0.45436 0.45436 0.5 0.5 0.5 0.54564 0.54564 0.54564 0.554867 0.554867 0.554867 0.564528 0.564528 0.564528 0.573435 0.573435 0.573435 0.581452 0.581452 0.581452 0.588587 0.588587 0.588587 0.594933 0.594933 0.594933 0.600619 0.600619 0.600619 0.605775 0.605775 0.605775 0.610518 0.610518 0.610518 0.614948 0.614948 0.614948 0.619147 0.619147 0.619147 0.623181 0.623181 0.623181 0.627101 0.627101 0.627101 0.630952 0.630952 0.630952 0.634768 0.634768 0.634768 0.638576 0.638576 0.638576 0.6424 0.6424 0.6424 0.646258 0.646258 0.646258 0.650166 0.650166 0.650166 0.654136 0.654136 0.654136 0.65818 0.65818 0.65818 0.662306 0.662306 0.662306 0.666523 0.666523 0.666523 0.670836 0.670836 0.670836 0.690118 0.690118 0.690118 0.704708 0.704708 0.704708 0.720964 0.720964 0.720964 0.738885 0.738885 0.738885 0.758471 0.758471 0.758471 0.779723 0.779723 0.779723 0.80264 0.80264 0.80264 0.827222 0.827222 0.827222 0.85347 0.85347 0.85347 0.881383 0.881383 0.881383 0.910962 0.910962 0.910962 0.942205 0.942205 0.942205 1 1 1 1
  arc A246 (19.4256, 43.3472) -> (20.4266, 43.933) centre (0.0435, 77.6158) ccw
  spline S45 degree 3 poles (22.9014, 45.5609) (22.7897, 45.6365) (22.679, 45.7136) (22.5697, 45.7925) (22.5105, 45.8352) (22.4518, 45.8783) (22.3934, 45.922) (22.3382, 45.9634) (22.2833, 46.0052) (22.2288, 46.0476) (22.1773, 46.0875) (22.1262, 46.1279) (22.0755, 46.1688) (22.0278, 46.2072) (21.9804, 46.2461) (21.9334, 46.2854) (21.8894, 46.3221) (21.8457, 46.3593) (21.8023, 46.3968) (21.7619, 46.4319) (21.7218, 46.4672) (21.682, 46.5029) (21.6451, 46.5361) (21.6085, 46.5695) (21.5722, 46.6033) (21.5387, 46.6344) (21.5055, 46.6658) (21.4726, 46.6976) (21.4425, 46.7266) (21.4126, 46.7559) (21.3831, 46.7854) (21.3562, 46.8122) (21.3296, 46.8393) (21.3033, 46.8666) (21.2796, 46.891) (21.2561, 46.9157) (21.2329, 46.9406) (21.2023, 46.9736) (21.1721, 47.0069) (21.1422, 47.0406) (21.1355, 47.0481) (21.1288, 47.0556) (21.1221, 47.0631) (21.1155, 47.0704) (21.1088, 47.0776) (21.102, 47.0847) (21.0954, 47.0918) (21.0888, 47.0987) (21.0821, 47.1056) (21.0755, 47.1124) (21.0688, 47.1191) (21.0621, 47.1257) (21.0555, 47.1322) (21.0489, 47.1387) (21.0422, 47.1451) (21.0356, 47.1513) (21.0289, 47.1575) (21.0221, 47.1637) (21.0155, 47.1697) (21.0087, 47.1757) (21.0019, 47.1816) (20.9952, 47.1875) (20.9884, 47.1932) (20.9815, 47.1989) (20.9746, 47.2045) (20.9677, 47.2101) (20.9607, 47.2156) (20.9537, 47.221) (20.9465, 47.2264) (20.9394, 47.2317) (20.9321, 47.237) (20.9248, 47.2421) (20.9173, 47.2472) (20.9098, 47.2524) (20.9021, 47.2574) (20.8944, 47.2622) (20.8864, 47.2672) (20.8783, 47.2721) (20.8702, 47.2768) (20.8617, 47.2816) (20.853, 47.2863) (20.8443, 47.2908) (20.8351, 47.2955) (20.8258, 47.3) (20.8164, 47.3042) (20.8062, 47.3087) (20.796, 47.3129) (20.7856, 47.3168) (20.7744, 47.321) (20.763, 47.3249) (20.7514, 47.3283) (20.7387, 47.3321) (20.7258, 47.3354) (20.7129, 47.3381) (20.6984, 47.3412) (20.6837, 47.3435) (20.669, 47.3452) (20.6524, 47.3471) (20.6358, 47.348) (20.6191, 47.348) (20.6004, 47.348) (20.5817, 47.3469) (20.5631, 47.3445) (20.5425, 47.3418) (20.5221, 47.3376) (20.502, 47.332) (20.4803, 47.3259) (20.459, 47.3181) (20.4386, 47.3085) (20.4192, 47.2993) (20.4005, 47.2884) (20.3821, 47.2772) (20.291, 47.2218) (20.2049, 47.1589) (20.1159, 47.1004) (20.027, 47.0419) (19.9352, 46.9877) (19.8482, 46.926) (19.8307, 46.9135) (19.8133, 46.9007) (19.7971, 46.8865) (19.7802, 46.8716) (19.7646, 46.8552) (19.7504, 46.8376) (19.7373, 46.8214) (19.7254, 46.8043) (19.7148, 46.7864) (19.7052, 46.7703) (19.6967, 46.7536) (19.6893, 46.7364) (19.6827, 46.7211) (19.677, 46.7055) (19.6722, 46.6895) (19.6679, 46.6753) (19.6643, 46.661) (19.6613, 46.6464) (19.6587, 46.6334) (19.6566, 46.6203) (19.655, 46.6071) (19.6536, 46.5952) (19.6526, 46.5832) (19.6521, 46.5712) (19.6515, 46.5601) (19.6514, 46.549) (19.6515, 46.538) (19.6516, 46.5276) (19.6521, 46.5173) (19.6527, 46.507) (19.6534, 46.4972) (19.6543, 46.4874) (19.6554, 46.4777) (19.6564, 46.4683) (19.6577, 46.459) (19.6591, 46.4497) (19.6605, 46.4407) (19.6621, 46.4317) (19.6638, 46.4227) (19.6655, 46.4138) (19.6674, 46.405) (19.6694, 46.3963) (19.6714, 46.3876) (19.6735, 46.379) (19.6757, 46.3703) (19.678, 46.3617) (19.6803, 46.3532) (19.6828, 46.3446) (19.6853, 46.3361) (19.6879, 46.3275) (19.6906, 46.319) (19.6933, 46.3104) (19.6961, 46.3019) (19.699, 46.2934) (19.702, 46.2847) (19.705, 46.2762) (19.7082, 46.2676) (19.7114, 46.2589) (19.7147, 46.2502) (19.7181, 46.2416) (19.7215, 46.2328) (19.725, 46.2241) (19.7286, 46.2153) (19.7323, 46.2064) (19.736, 46.1976) (19.7399, 46.1887) (19.7438, 46.1797) (19.7478, 46.1707) (19.7518, 46.1618) (19.756, 46.1526) (19.7603, 46.1435) (19.7645, 46.1344) (19.7836, 46.0936) (19.8022, 46.0527) (19.8204, 46.0115) (19.8341, 45.9803) (19.8474, 45.949) (19.8605, 45.9176) (19.8751, 45.8825) (19.8894, 45.8474) (19.9034, 45.8122) (19.9189, 45.7733) (19.9339, 45.7343) (19.9486, 45.6951) (19.9647, 45.6524) (19.9804, 45.6094) (19.9958, 45.5664) (20.0124, 45.5197) (20.0286, 45.4728) (20.0444, 45.4258) (20.0615, 45.3751) (20.0781, 45.3243) (20.0942, 45.2733) (20.1115, 45.2186) (20.1283, 45.1637) (20.1447, 45.1087) (20.1621, 45.05) (20.179, 44.9912) (20.1955, 44.9321) (20.2129, 44.8694) (20.2298, 44.8065) (20.2461, 44.7434) (20.2634, 44.6766) (20.2801, 44.6096) (20.2962, 44.5425) (20.3132, 44.4716) (20.3296, 44.4006) (20.3453, 44.3294) (20.3745, 44.1977) (20.4015, 44.0655) (20.4266, 43.933) knots 0 0 0 0 0.057795 0.057795 0.057795 0.089038 0.089038 0.089038 0.118617 0.118617 0.118617 0.14653 0.14653 0.14653 0.172778 0.172778 0.172778 0.19736 0.19736 0.19736 0.220277 0.220277 0.220277 0.241529 0.241529 0.241529 0.261115 0.261115 0.261115 0.279036 0.279036 0.279036 0.295292 0.295292 0.295292 0.309882 0.309882 0.309882 0.329164 0.329164 0.329164 0.333477 0.333477 0.333477 0.337694 0.337694 0.337694 0.34182 0.34182 0.34182 0.345864 0.345864 0.345864 0.349834 0.349834 0.349834 0.353742 0.353742 0.353742 0.3576 0.3576 0.3576 0.361424 0.361424 0.361424 0.365232 0.365232 0.365232 0.369048 0.369048 0.369048 0.372899 0.372899 0.372899 0.376819 0.376819 0.376819 0.380853 0.380853 0.380853 0.385052 0.385052 0.385052 0.389482 0.389482 0.389482 0.394225 0.394225 0.394225 0.399381 0.399381 0.399381 0.405067 0.405067 0.405067 0.411413 0.411413 0.411413 0.418548 0.418548 0.418548 0.426565 0.426565 0.426565 0.435472 0.435472 0.435472 0.445133 0.445133 0.445133 0.45436 0.45436 0.45436 0.5 0.5 0.5 0.54564 0.54564 0.54564 0.554867 0.554867 0.554867 0.564528 0.564528 0.564528 0.573435 0.573435 0.573435 0.581452 0.581452 0.581452 0.588587 0.588587 0.588587 0.594933 0.594933 0.594933 0.600619 0.600619 0.600619 0.605775 0.605775 0.605775 0.610518 0.610518 0.610518 0.614948 0.614948 0.614948 0.619147 0.619147 0.619147 0.623181 0.623181 0.623181 0.627101 0.627101 0.627101 0.630952 0.630952 0.630952 0.634768 0.634768 0.634768 0.638576 0.638576 0.638576 0.6424 0.6424 0.6424 0.646258 0.646258 0.646258 0.650166 0.650166 0.650166 0.654136 0.654136 0.654136 0.65818 0.65818 0.65818 0.662306 0.662306 0.662306 0.666523 0.666523 0.666523 0.670836 0.670836 0.670836 0.690118 0.690118 0.690118 0.704708 0.704708 0.704708 0.720964 0.720964 0.720964 0.738885 0.738885 0.738885 0.758471 0.758471 0.758471 0.779723 0.779723 0.779723 0.80264 0.80264 0.80264 0.827222 0.827222 0.827222 0.85347 0.85347 0.85347 0.881383 0.881383 0.881383 0.910962 0.910962 0.910962 0.942205 0.942205 0.942205 1 1 1 1
  arc A247 (22.9014, 45.5609) -> (23.8357, 46.2482) centre (0.0435, 77.6158) ccw